Autodesk Fusion 360 part; units mm, degrees
(part 5 of 5)
sketch "Sketch1 (28)" plane through (0, 0, 0) normal (0, 0, 1) x (1, 0, 0) in component "main-switchbody (9)"
  line L0 (0, 0) -> (0, 20) construction
  line L1 (0, 20) -> (20, 20) construction
  line L2 (20, 20) -> (20, 0) construction
  line L3 (20, 0) -> (0, 0) construction
  line L4 (0, 0) -> (20, 20) construction
  line L5 (20, 0) -> (0, 20) construction
  line L6 (10, 0) -> (18.9, 0) construction
  line L7 (10, 10) -> (18.9, 10) construction
  line L8 (18.9, 10) -> (18.9, 18.9) construction
  line L9 (18.9, 18.9) -> (1.1, 18.9) construction
  line L10 (1.1, 18.9) -> (1.1, 1.1) construction
  line L11 (1.1, 1.1) -> (18.9, 1.1) construction
  line L12 (18.9, 1.1) -> (18.9, 18.9) construction
  line L13 (10, 10) -> (3.05, 10) construction
  line L14 (3.05, 10) -> (3.05, 16.95) construction
  line L15 (3.05, 16.95) -> (16.95, 16.95) construction
  line L16 (16.95, 16.95) -> (16.95, 3.05) construction
  line L17 (16.95, 3.05) -> (3.05, 3.05) construction
  line L18 (3.05, 3.05) -> (3.05, 16.95) construction
  line L19 (3.05, 3.05) -> (0, 3.05) construction
  line L20 (3.05, 3.05) -> (3.05, 0) construction
  line L21 (16.95, 3.05) -> (20, 3.05) construction
  line L22 (16.95, 16.95) -> (20, 16.95) construction
  line L23 (16.95, 16.95) -> (16.95, 20) construction
  line L24 (3.05, 16.95) -> (3.05, 20) construction
  line L25 (3.05, 16.95) -> (0, 16.95) construction
  line L26 (3.05, 18.9) -> (6.05, 18.9) construction
  line L27 (6.05, 18.9) -> (6.05, 20) construction
  line L28 (16.95, 18.9) -> (13.95, 18.9) construction
  line L29 (13.95, 18.9) -> (13.95, 20) construction
  line L30 (16.95, 3.05) -> (16.95, 0) construction
  line L31 (16.95, 1.1) -> (13.95, 1.1) construction
  line L32 (13.95, 1.1) -> (13.95, 0) construction
  line L33 (3.05, 1.1) -> (6.05, 1.1) construction
  line L34 (6.05, 1.1) -> (6.05, 0) construction
  line L35 (0, 20) -> (20, 20) construction
  line L36 (20, 20) -> (20, 0) construction
  line L37 (20, 0) -> (0, 0) construction
  line L38 (0, 0) -> (0, 20) construction
  line L39 (0, 20) -> (20, 20)
  line L40 (20, 20) -> (20, 0)
  line L41 (20, 0) -> (0, 0)
  line L42 (0, 0) -> (0, 20)
  line L43 (16.95, 3.05) -> (3.05, 3.05)
  line L44 (3.05, 3.05) -> (3.05, 16.95)
  line L45 (3.05, 16.95) -> (16.95, 16.95)
  line L46 (16.95, 16.95) -> (16.95, 3.05)
  line L47 (3.05, 1.1) -> (6.05, 1.1)
  line L48 (6.05, 1.1) -> (6.05, 0)
  line L49 (6.05, 0) -> (3.05, 0)
  line L50 (3.05, 0) -> (3.05, 1.1)
  line L51 (13.95, 1.1) -> (16.95, 1.1)
  line L52 (16.95, 1.1) -> (16.95, 0)
  line L53 (16.95, 0) -> (13.95, 0)
  line L54 (13.95, 0) -> (13.95, 1.1)
  line L55 (13.95, 20) -> (16.95, 20)
  line L56 (16.95, 20) -> (16.95, 18.9)
  line L57 (16.95, 18.9) -> (13.95, 18.9)
  line L58 (13.95, 18.9) -> (13.95, 20)
  line L59 (3.05, 20) -> (6.05, 20)
  line L60 (6.05, 20) -> (6.05, 18.9)
  line L61 (6.05, 18.9) -> (3.05, 18.9)
  line L62 (3.05, 18.9) -> (3.05, 20)
  line L63 (1.1, 10) -> (1.1, 12)
  line L64 (1.1, 10) -> (1.1, 8)
  line L65 (1.1, 8) -> (-1.9, 8)
  line L66 (-1.9, 8) -> (1.1, 8)
  line L67 (1.1, 8) -> (1.1, 12)
  line L68 (1.1, 12) -> (-1.9, 12)
  line L69 (-1.9, 12) -> (-1.9, 8)
  line L70 (3.05, 10) -> (3.05, 7.5) construction
  line L71 (3.05, 7.5) -> (2.55, 7.5) construction
  line L72 (2.55, 7.5) -> (2.55, 12.5) construction
  line L73 (2.55, 12.5) -> (3.05, 12.5085) construction
  line L74 (3.05, 12.5085) -> (3.05, 7.5) construction
  line L75 (2.55, 12.5) -> (16.95, 12.5) construction
  line L76 (16.95, 12.5) -> (17.45, 12.5) construction
  line L77 (17.45, 12.5) -> (17.45, 7.5) construction
  line L78 (17.45, 7.5) -> (16.95, 7.5) construction
  line L79 (16.95, 7.5) -> (16.95, 12.5) construction
  line L80 (17.45, 7.5) -> (16.95, 7.5)
  line L81 (16.95, 7.5) -> (16.95, 12.5)
  line L82 (16.95, 12.5) -> (17.45, 12.5)
  line L83 (17.45, 12.5) -> (17.45, 7.5)
  line L84 (3.05, 7.5) -> (2.55, 7.5)
  line L85 (2.55, 7.5) -> (2.55, 12.5)
  line L86 (2.55, 12.5) -> (3.05, 12.5)
  line L87 (3.05, 12.5) -> (3.05, 7.5)
  dimension "d1_9" = 20
  dimension "d2_9" = 20
  dimension "d3_9" = 8.9
  dimension "d4_9" = 8.9
  dimension "d5_9" = 8.9
  dimension "d6_9" = 17.8
  dimension "d7_9" = 17.8
  dimension "d8_9" = 6.95
  dimension "d9_9" = 6.95
  dimension "d10_9" = 13.9
  dimension "d11_9" = 13.9
  dimension "d12_9" = 13.9
  dimension "d13_9" = 3
  dimension "d14_9" = 3
  dimension "d15_9" = 3
  dimension "d16_9" = 3
  dimension "d21_15" = 3
  dimension "d58_15" = 2.5
  dimension "d59_15" = 0.5
  dimension "d60_15" = 5
  dimension "d61_15" = 0.5
  dimension "d62_15" = 5
  constraint coincident L0.start L3.end
  constraint vertical L0
  constraint perpendicular L0 L1
  constraint perpendicular L1 L2
  constraint perpendicular L0 L3
  constraint midpoint L3 L6.start
  constraint parallel L3 L6
  constraint midpoint L4 L7.start
  constraint parallel L6 L7
  constraint perpendicular L7 L8
  constraint perpendicular L8 L9
  constraint perpendicular L9 L10
  constraint coincident L5 L11.end
  constraint perpendicular L10 L11
  constraint perpendicular L12 L13
  constraint perpendicular L13 L14
  constraint perpendicular L14 L15
  constraint perpendicular L7 L16
  constraint perpendicular L16 L17
  constraint coincident L0 L19.end
  constraint perpendicular L0 L19
  constraint coincident L3 L20.end
  constraint perpendicular L3 L20
  constraint coincident L2 L21.end
  constraint perpendicular L2 L21
  constraint coincident L2 L22.end
  constraint perpendicular L2 L22
  constraint coincident L1 L23.end
  constraint perpendicular L1 L23
  constraint coincident L1 L24.end
  constraint perpendicular L1 L24
  constraint coincident L0 L25.end
  constraint perpendicular L0 L25
  constraint coincident L24 L26.start
  constraint coincident L9 L26.start
  constraint coincident L9 L26.end
  constraint coincident L1 L27.end
  constraint perpendicular L1 L27
  constraint coincident L9 L28.start
  constraint coincident L23 L28.start
  constraint perpendicular L23 L28
  constraint coincident L1 L29.end
  constraint perpendicular L1 L29
  constraint coincident L6 L30.end
  constraint coincident L30 L31.start
  constraint coincident L11 L31.start
  constraint perpendicular L30 L31
  constraint coincident L6 L32.end
  constraint coincident L11 L33.start
  constraint coincident L20 L33.start
  constraint perpendicular L20 L33
  constraint coincident L3 L34.end
  constraint perpendicular L3 L34
  constraint horizontal L35
  constraint vertical L36
  constraint horizontal L37
  constraint vertical L38
  constraint horizontal L39
  constraint vertical L40
  constraint horizontal L41
  constraint vertical L42
  constraint horizontal L43
  constraint vertical L44
  constraint horizontal L45
  constraint vertical L46
  constraint horizontal L47
  constraint vertical L48
  constraint horizontal L49
  constraint vertical L50
  constraint horizontal L51
  constraint vertical L52
  constraint horizontal L53
  constraint vertical L54
  constraint horizontal L55
  constraint vertical L56
  constraint horizontal L57
  constraint vertical L58
  constraint horizontal L59
  constraint vertical L60
  constraint horizontal L61
  constraint vertical L62
  constraint midpoint L10 L63.start
  constraint coincident L10 L63.end
  constraint parallel L10 L63
  constraint coincident L10 L64.end
  constraint perpendicular L0 L65
  constraint horizontal L66
  constraint vertical L67
  constraint horizontal L68
  constraint vertical L69
  constraint perpendicular L13 L70
  constraint perpendicular L70 L71
  constraint perpendicular L71 L72
  constraint coincident L14 L73.end
  constraint perpendicular L71 L74
  constraint coincident L16 L75.end
  constraint perpendicular L16 L75
  constraint perpendicular L16 L76
  constraint perpendicular L76 L77
  constraint coincident L16 L78.end
  constraint perpendicular L16 L78
  constraint horizontal L80
  constraint vertical L81
  constraint horizontal L82
  constraint vertical L83
  constraint horizontal L84
  constraint vertical L85
  constraint horizontal L86
  constraint vertical L87
  measures "d1_9" distance of L0.start L0.end
  measures "d2_9" distance of L0.end L1.end
  measures "d3_9" distance of L6.start L6.end
  measures "d4_9" distance of L7.start L7.end
  measures "d5_9" distance of L7.end L8.end
  measures "d6_9" distance of L8.end L9.end
  measures "d7_9" distance of L9.end L10.end
  measures "d8_9" distance of L7.start L13.end
  measures "d9_9" distance of L13.end L14.end
  measures "d10_9" distance of L14.end L15.end
  measures "d11_9" distance of L15.end L16.end
  measures "d12_9" distance of L16.end L17.end
  measures "d13_9" distance of L26.start L26.end
  measures "d14_9" distance of L28.start L28.end
  measures "d15_9" distance of L31.start L31.end
  measures "d16_9" distance of L33.start L33.end
  measures "d21_15" distance of L64.end L65.end
  measures "d58_15" distance of L13.end L70.end
  measures "d59_15" distance of L70.end L71.end
  measures "d60_15" distance of L71.end L72.end
  measures "d61_15" distance of L75.end L76.end
  measures "d62_15" distance of L76.end L77.end
extrude "Extrude3'''''''''''" add sketch "Sketch1 (28)" along normal blind 7.5 separate body contours L42 L63 L64 L65 L66 L67 L68 | L42 L65 L66 L68 L69 makes body 43 in component "main-switchbody (9)"
extrude "Extrude2'''''''''''" add sketch "Sketch1 (28)" along normal blind 4 separate body contours L39 L40 L41 L42 L47 L48 L50 L51 L52 L54 L56 L57 L58 L60 L61 L62 L63 L64 L65 L66 L67 L68 | L42 L63 L64 L65 L66 L67 L68 | L46 L80 L81 L82 L83 | L44 L84 L85 L86 L87 makes body 44 in component "main-switchbody (9)"
extrude "Extrude1'''''''''''''''''" add sketch "Sketch1 (28)" along normal blind 6 separate body contours L39 L59 L60 L61 L62 | L39 L55 L56 L57 L58 | L41 L47 L48 L49 L50 | L41 L51 L52 L53 L54 makes body 45 at (4.05, 1.1, 2) makes body 46 at (5.05, 20, 4) makes body 47 at (14.95, 1.1, 2) makes body 48 at (14.95, 20, 2) in component "main-switchbody (9)"
extrude "Extrude4'''''" cut sketch "Sketch1 (28)" along normal blind 2 contours L42 L65 L66 L68 L69 bodies 43 in component "main-switchbody (9)"
sketch "Sketch2 (22)" plane through (1.1, 0, 0) normal (1, 0, 0) x (0, 1, 0) in component "main-switchbody (9)"
  line L0 (8, 0) -> (12, 0)
  line L1 (12, 0) -> (12, 7.5)
  line L2 (12, 7.5) -> (8, 7.5)
  line L3 (8, 7.5) -> (8, 0)
  line L4 (8, 7.5) -> (8, 4) construction
  line L5 (8, 4) -> (12, 4) construction
  line L6 (12, 4) -> (12, 7.5) construction
  line L7 (12, 7.5) -> (8, 7.5) construction
  line L8 (8, 7.5) -> (8, 5.75) construction
  line L9 (8, 5.75) -> (12, 5.75) construction
  line L10 (8, 7.5) -> (12, 7.5)
  line L11 (12, 7.5) -> (12, 5.75)
  line L12 (12, 5.75) -> (8, 5.75)
  line L13 (8, 5.75) -> (8, 7.5)
  dimension "d26_15" = 1.75
  constraint coincident L2.end L3.start
  constraint coincident L3 L4.end
  constraint perpendicular L2 L4
  constraint coincident L1 L5.end
  constraint perpendicular L1 L5
  constraint coincident L1.end L2.start
  constraint perpendicular L2 L6
  constraint perpendicular L5 L8
  constraint midpoint L6 L9.end
  constraint horizontal L10
  constraint vertical L11
  constraint horizontal L12
  constraint vertical L13
  measures "d26_15" distance of L2.end L8.end
extrude "Extrude5'''''" add sketch "Sketch2 (22)" along normal blind 1 contours L1 L2 L3 L10 L11 L12 L13 bodies 43 in component "main-switchbody (9)"
extrude "Extrude6'''''" cut 1 faces at (-1.9, 10.6667, 3.8333) along direction (1, 0, 0) blind 1 on bodies 43 bodies 43 in component "main-switchbody (9)"
sketch "Sketch3 (6)" plane through (0, 18.9, 0) normal (0, -1, 0) x (1, 0, 0) in component "main-switchbody (9)"
  line L0 (3.05, 0) -> (6.05, 0)
  line L1 (6.05, 0) -> (6.05, 6)
  line L2 (6.05, 6) -> (3.05, 6)
  line L3 (3.05, 6) -> (3.05, 0)
  line L4 (3.05, 6) -> (3.05, 4) construction
  line L5 (6.05, 4) -> (6.05, 6) construction
  line L6 (3.05, 6) -> (3.05, 4.5) construction
  line L7 (6.05, 6) -> (6.05, 4.5) construction
  arc A0 (6.05, 4.5) -> (3.05, 4.5) centre (4.55, 4.5) ccw construction
  arc A1 (6.05, 4.5) -> (3.05, 4.5) centre (4.55, 4.5) ccw
  dimension "d31_15" = 1.5
  dimension "d32_15" = 1.5
  constraint coincident L2.end L3.start
  constraint coincident L3 L4.end
  constraint perpendicular L2 L4
  constraint coincident L1 L5.start
  constraint coincident L1.end L2.start
  constraint perpendicular L2 L5
  constraint perpendicular L2 L6
  constraint perpendicular L2 L7
  constraint tangent L2 A0
  constraint tangent L2 A1
  measures "d31_15" distance of L2.end L6.end
  measures "d32_15" distance of L1.end L7.end
extrude "Extrude7'''''" cut sketch "Sketch3 (6)" against normal blind 1.1 contours L2 L3 A1 | L1 L2 A1 bodies 46 in component "main-switchbody (9)"
sketch "Sketch4 (6)" plane through (0, 0, 0) normal (0, -1, 0) x (1, 0, 0) in component "main-switchbody (9)"
  line L0 (3.05, 0) -> (6.05, 0)
  line L1 (6.05, 0) -> (6.05, 6)
  line L2 (6.05, 6) -> (3.05, 6)
  line L3 (3.05, 6) -> (3.05, 0)
  line L4 (3.05, 6) -> (3.05, 4.5) construction
  line L5 (6.05, 6) -> (6.05, 4.5) construction
  arc A0 (6.05, 4.5) -> (3.05, 4.5) centre (4.55, 4.5) ccw
  constraint coincident L2.end L3.start
  constraint coincident L3 L4.end
  constraint perpendicular L2 L4
  constraint coincident L1.end L2.start
  constraint coincident L1 L5.end
  constraint perpendicular L2 L5
  constraint tangent L2 A0
extrude "Extrude8'''''" cut sketch "Sketch4 (6)" against normal blind 1.1 contours L2 L3 A0 | L1 L2 A0 bodies 45 in component "main-switchbody (9)"
sketch "Sketch5 (6)" plane through (0, 0, 0) normal (0, -1, 0) x (1, 0, 0) in component "main-switchbody (9)"
  line L0 (13.95, 0) -> (16.95, 0)
  line L1 (16.95, 0) -> (16.95, 6)
  line L2 (16.95, 6) -> (13.95, 6)
  line L3 (13.95, 6) -> (13.95, 0)
  line L4 (13.95, 6) -> (13.95, 4.5) construction
  line L5 (16.95, 6) -> (16.95, 4.5) construction
  arc A0 (16.95, 4.5) -> (13.95, 4.5) centre (15.45, 4.5) ccw
  constraint coincident L2.end L3.start
  constraint coincident L3 L4.end
  constraint perpendicular L2 L4
  constraint coincident L1.end L2.start
  constraint coincident L1 L5.end
  constraint perpendicular L2 L5
  constraint tangent L2 A0
extrude "Extrude9'''''" cut sketch "Sketch5 (6)" against normal blind 1.1 contours L2 L3 A0 | L1 L2 A0 bodies 47 in component "main-switchbody (9)"
sketch "Sketch6 (6)" plane through (0, 18.9, 0) normal (0, -1, 0) x (1, 0, 0) in component "main-switchbody (9)"
  line L0 (13.95, 0) -> (16.95, 0)
  line L1 (16.95, 0) -> (16.95, 6)
  line L2 (16.95, 6) -> (13.95, 6)
  line L3 (13.95, 6) -> (13.95, 0)
  line L4 (13.95, 6) -> (13.95, 4.5) construction
  line L5 (16.95, 6) -> (16.95, 4.5) construction
  arc A0 (16.95, 4.5) -> (13.95, 4.5) centre (15.45, 4.5) ccw
  constraint coincident L2.end L3.start
  constraint coincident L3 L4.end
  constraint perpendicular L2 L4
  constraint coincident L1.end L2.start
  constraint coincident L1 L5.end
  constraint perpendicular L2 L5
  constraint tangent L2 A0
extrude "Extrude10'''''" cut sketch "Sketch6 (6)" against normal blind 1.1 contours L2 L3 A0 | L1 L2 A0 bodies 48 in component "main-switchbody (9)"
sketch "Sketch7 (6)" plane through (0, 0, 4) normal (0, 0, 1) x (-1, 0, 0) in component "main-switchbody (9)"
  line L0 (-3.05, -16.95) -> (-16.95, -16.95)
  line L1 (-16.95, -16.95) -> (-16.95, -3.05)
  line L2 (-16.95, -3.05) -> (-3.05, -3.05)
  line L3 (-3.05, -3.05) -> (-3.05, -16.95)
  line L4 (-6.05, -20) -> (-6.05, -18.9)
  line L5 (-6.05, -18.9) -> (-3.05, -18.9)
  line L6 (-3.05, -18.9) -> (-3.05, -20)
  line L7 (-3.05, -20) -> (0, -20)
  line L8 (0, -20) -> (0, 0)
  line L9 (0, 0) -> (-3.05, 0)
  line L10 (-3.05, 0) -> (-3.05, -1.1)
  line L11 (-3.05, -1.1) -> (-6.05, -1.1)
  line L12 (-6.05, -1.1) -> (-6.05, 0)
  line L13 (-6.05, 0) -> (-13.95, 0)
  line L14 (-13.95, 0) -> (-13.95, -1.1)
  line L15 (-13.95, -1.1) -> (-16.95, -1.1)
  line L16 (-16.95, -1.1) -> (-16.95, 0)
  line L17 (-16.95, 0) -> (-20, 0)
  line L18 (-20, 0) -> (-20, -20)
  line L19 (-20, -20) -> (-16.95, -20)
  line L20 (-16.95, -20) -> (-16.95, -18.9)
  line L21 (-16.95, -18.9) -> (-13.95, -18.9)
  line L22 (-13.95, -18.9) -> (-13.95, -20)
  line L23 (-13.95, -20) -> (-6.05, -20)
  line L24 (-20, -10) -> (-20, -11.5) construction
  line L25 (-20, -10) -> (-20, -8.5) construction
  line L26 (-20, -8.5) -> (-19, -8.5) construction
  line L27 (-19, -8.5) -> (-19, -11.5) construction
  line L28 (-19, -11.5) -> (-20, -11.5) construction
  line L29 (-20, -11.5) -> (-21, -11.5) construction
  line L30 (-21, -11.5) -> (-21, -8.5) construction
  line L31 (-21, -8.5) -> (-20, -8.5) construction
  line L32 (-19, -11.5) -> (-21, -11.5)
  line L33 (-21, -11.5) -> (-21, -8.5)
  line L34 (-21, -8.5) -> (-19, -8.5)
  line L35 (-19, -8.5) -> (-19, -11.5)
  dimension "d41_15" = 1.5
  dimension "d42_15" = 1
  constraint midpoint L18 L24.start
  constraint parallel L18 L24
  constraint coincident L18 L25.end
  constraint parallel L18 L25
  constraint perpendicular L25 L26
  constraint perpendicular L26 L27
  constraint perpendicular L24 L29
  constraint perpendicular L29 L30
  constraint horizontal L32
  constraint vertical L33
  constraint horizontal L34
  constraint vertical L35
  measures "d41_15" distance of L24.start L24.end
  measures "d42_15" distance of L24.end L29.end
extrude "Extrude11'''''" add sketch "Sketch7 (6)" along normal blind 3 contours L18 L32 L33 L34 | L18 L32 L34 L35 bodies 44 in component "main-switchbody (9)"
extrude "Extrude12'''''" add 1 faces at (20, 8.5, 6) along direction (0, -1, 0) blind 0.5 on bodies 44 bodies 44 in component "main-switchbody (9)"
extrude "Extrude13'''''" add 1 faces at (20, 11.5, 6) along direction (0, 1, 0) blind 0.5 on bodies 44 bodies 44 in component "main-switchbody (9)"
extrude "Extrude14'''''" add 1 faces at (20.3333, 10.6667, 7) along direction (0, 0, 1) blind 0.75 on bodies 44 bodies 44 in component "main-switchbody (9)"
sketch "Sketch8 (6)" plane through (0, 0, 4) normal (0, 0, -1) x (1, 0, 0) in component "main-switchbody (9)"
  line L0 (20, -8) -> (20, -12)
  line L1 (20, -12) -> (21, -12)
  line L2 (21, -12) -> (21, -8)
  line L3 (21, -8) -> (20, -8)
  line L4 (20, -12) -> (20, -8)
  constraint coincident L0.end L1.start
  constraint coincident L0.start L3.end
extrude "Extrude15'''''" add sketch "Sketch8 (6)" along normal blind 2 bodies 44 in component "main-switchbody (9)"
sketch "Sketch9 (11)" plane through (19, 0, 0) normal (-1, 0, 0) x (0, -1, 0) in component "main-switchbody (9)"
  line L0 (-12, 4) -> (-8, 4)
  line L1 (-8, 4) -> (-8, 7.75)
  line L2 (-8, 7.75) -> (-12, 7.75)
  line L3 (-12, 7.75) -> (-12, 4)
  line L4 (-12, 7.75) -> (-12, 5.75) construction
  line L5 (-12, 5.75) -> (-8, 5.75) construction
  line L6 (-12, 7.75) -> (-8, 7.75)
  line L7 (-8, 7.75) -> (-8, 5.75)
  line L8 (-8, 5.75) -> (-12, 5.75)
  line L9 (-12, 5.75) -> (-12, 7.75)
  dimension "d53_15" = 2
  constraint coincident L2.end L3.start
  constraint perpendicular L2 L4
  constraint coincident L1 L5.end
  constraint perpendicular L1 L5
  constraint horizontal L6
  constraint vertical L7
  constraint horizontal L8
  constraint vertical L9
  measures "d53_15" distance of L2.end L4.end
extrude "Extrude16'''''" add sketch "Sketch9 (11)" along normal blind 0.5 contours L1 L2 L3 L6 L7 L8 L9 bodies 44 in component "main-switchbody (9)"
extrude "Extrude17'''''" cut 1 faces at (2.1, 9.3333, 6.9167) along direction (-1, 0, 0) blind 0.3 on bodies 43 bodies 43 in component "main-switchbody (9)"
extrude "Extrude18'''''" cut sketch "Sketch1 (28)" along normal blind 2.7 contours L44 L84 L85 L86 L87 bodies 44 in component "main-switchbody (9)"
extrude "Extrude19'''''" cut sketch "Sketch1 (28)" along normal blind 2.7 contours L46 L80 L81 L82 L83 bodies 44 in component "main-switchbody (9)"
extrude "Extrude20'''''" add sketch "Sketch1 (28)" against normal blind 0.2 contours L39 L40 L41 L42 L47 L48 L50 L51 L52 L54 L56 L57 L58 L60 L61 L62 L63 L64 L65 L66 L67 L68 | L39 L59 L60 L61 L62 | L42 L63 L64 L65 L66 L67 L68 | L39 L55 L56 L57 L58 | L41 L47 L48 L49 L50 | L41 L51 L52 L53 L54 bodies 43 44 45 46 47 48 in component "main-switchbody (9)"
fillet "Fillet1'''''" radius 1 2 edges at (21, 10, 7.75) (-0.9, 10, 7.5) on bodies 43 44 in component "main-switchbody (9)"
extrude "Extrude21'''''" add 1 faces at (2.8833, 9.1667, 2.7) along direction (0, 0, -1) blind 2.9 on bodies 43 bodies 43 in component "main-switchbody (9)"
extrude "Extrude22'''''" add 1 faces at (17.1167, 10.8333, 2.7) along direction (0, 0, -1) blind 2.9 on bodies 43 bodies 43 in component "main-switchbody (9)"
sketch "Sketch10 (6)" plane through (0, 0, 4) normal (0, 0, 1) x (-1, 0, 0) in component "main-switchbody (9)"
  line L0 (-3.05, -16.95) -> (-16.95, -16.95)
  line L1 (-16.95, -16.95) -> (-16.95, -3.05)
  line L2 (-16.95, -3.05) -> (-3.05, -3.05)
  line L3 (-3.05, -3.05) -> (-3.05, -16.95)
  line L4 (0, -12) -> (-1.1, -12)
  line L5 (-1.1, -12) -> (-1.1, -8)
  line L6 (-1.1, -8) -> (0, -8)
  line L7 (0, -8) -> (0, 0)
  line L8 (0, 0) -> (-3.05, 0)
  line L9 (-3.05, 0) -> (-3.05, -1.1)
  line L10 (-3.05, -1.1) -> (-6.05, -1.1)
  line L11 (-6.05, -1.1) -> (-6.05, 0)
  line L12 (-6.05, 0) -> (-13.95, 0)
  line L13 (-13.95, 0) -> (-13.95, -1.1)
  line L14 (-13.95, -1.1) -> (-16.95, -1.1)
  line L15 (-16.95, -1.1) -> (-16.95, 0)
  line L16 (-16.95, 0) -> (-20, 0)
  line L17 (-20, 0) -> (-20, -8)
  line L18 (-20, -8) -> (-19, -8)
  line L19 (-19, -8) -> (-19, -12)
  line L20 (-19, -12) -> (-20, -12)
  line L21 (-20, -12) -> (-20, -20)
  line L22 (-20, -20) -> (-16.95, -20)
  line L23 (-16.95, -20) -> (-16.95, -18.9)
  line L24 (-16.95, -18.9) -> (-13.95, -18.9)
  line L25 (-13.95, -18.9) -> (-13.95, -20)
  line L26 (-13.95, -20) -> (-6.05, -20)
  line L27 (-6.05, -20) -> (-6.05, -18.9)
  line L28 (-6.05, -18.9) -> (-3.05, -18.9)
  line L29 (-3.05, -18.9) -> (-3.05, -20)
  line L30 (-3.05, -20) -> (0, -20)
  line L31 (0, -20) -> (0, -12)
  line L32 (-3.05, -10) -> (-3.05, -12.5) construction
  line L33 (-3.05, -12.5) -> (-3.05, -7.5) construction
  line L34 (-3.05, -7.5) -> (-2.55, -7.5) construction
  line L35 (-2.55, -7.5) -> (-3.05, -7.5) construction
  line L36 (-3.05, -7.5) -> (-3.05, -12.5) construction
  line L37 (-3.05, -12.5) -> (-2.55, -12.5) construction
  line L38 (-2.55, -12.5) -> (-2.55, -7.5) construction
  line L39 (-3.05, -12.5) -> (-16.95, -12.5) construction
  line L40 (-16.95, -12.5) -> (-16.95, -7.5) construction
  line L41 (-16.95, -7.5) -> (-17.45, -7.5) construction
  line L42 (-17.45, -7.5) -> (-16.95, -7.5) construction
  line L43 (-16.95, -7.5) -> (-16.95, -12.5) construction
  line L44 (-16.95, -12.5) -> (-17.45, -12.5) construction
  line L45 (-17.45, -12.5) -> (-17.45, -7.5) construction
  line L46 (-16.95, -12.5) -> (-17.45, -12.5)
  line L47 (-17.45, -12.5) -> (-17.45, -7.5)
  line L48 (-17.45, -7.5) -> (-16.95, -7.5)
  line L49 (-16.95, -7.5) -> (-16.95, -12.5)
  line L50 (-2.55, -12.5) -> (-3.05, -12.5)
  line L51 (-3.05, -12.5) -> (-3.05, -7.5)
  line L52 (-3.05, -7.5) -> (-2.55, -7.5)
  line L53 (-2.55, -7.5) -> (-2.55, -12.5)
  dimension "d75_9" = 5
  dimension "d76_9" = 0.5
  dimension "d77_9" = 0.5
  constraint midpoint L3 L32.start
  constraint coincident L3 L32.end
  constraint perpendicular L0 L32
  constraint parallel L3 L33
  constraint perpendicular L33 L34
  constraint horizontal L35
  constraint vertical L36
  constraint horizontal L37
  constraint vertical L38
  constraint coincident L1 L39.end
  constraint perpendicular L1 L39
  constraint coincident L1 L40.end
  constraint perpendicular L39 L40
  constraint perpendicular L40 L41
  constraint horizontal L42
  constraint vertical L43
  constraint horizontal L44
  constraint vertical L45
  constraint horizontal L46
  constraint vertical L47
  constraint horizontal L48
  constraint vertical L49
  constraint horizontal L50
  constraint vertical L51
  constraint horizontal L52
  constraint vertical L53
  measures "d75_9" distance of L32.end L33.end
  measures "d76_9" distance of L33.end L34.end
  measures "d77_9" distance of L40.end L41.end
extrude "Extrude23'''''" cut sketch "Sketch10 (6)" against normal blind 2.9 contours L3 L50 L51 L52 L53 | L1 L46 L47 L48 L49 bodies 43 in component "main-switchbody (9)"
extrude "Extrude24'''''" cut 2 faces at (4.8122, 18.9, 5.1079) (15.1626, 18.9, 5.4316) along direction (0, 1, 0) blind 0.25 on bodies 43 bodies 43 in component "main-switchbody (9)"
extrude "Extrude25'''''" cut 2 faces at (4.2822, 1.1, 5.1824) (15.2673, 1.1, 4.9654) along direction (0, -1, 0) blind 0.25 on bodies 43 bodies 43 in component "main-switchbody (9)"
extrude "Extrude26'''''" add 1 faces at (1.0167, 12.3167, -0.2) along direction (0, 0, -1) blind 1 on bodies 43 bodies 43 in component "main-switchbody (9)"
extrude "Extrude27'''''" cut 1 faces at (1.0167, 12.3167, -1.2) along direction (0, 0, 1) blind 0.2 on bodies 43 bodies 43 in component "main-switchbody (9)"
extrude "Extrude28'''''" cut 2 faces at (17.1167, 10.8333, 1.1) (2.8833, 9.1667, 1.1) along direction (0, 0, -1) blind 0.8 on bodies 43 bodies 43 in component "main-switchbody (9)"
extrude "Extrude29'''''" cut 1 faces at (18.8333, 9.3333, 5.75) along direction (0, 0, 1) blind 0.2 on bodies 43 bodies 43 in component "main-switchbody (9)"
extrude "Extrude30'''''" cut 1 faces at (1.3333, 10.6667, 5.75) along direction (0, 0, 1) blind 0.2 on bodies 43 bodies 43 in component "main-switchbody (9)"
sketch "Sketch1 (29)" plane through (0, 0, 0.0152) normal (0, 0, -1) x (1, 0, 0) in component "mxledbit-switchbody v10 (9)"
  line L0 (4.5419, -16.2374) -> (4.5419, -2.3374)
  line L1 (4.5419, -2.3374) -> (18.4419, -2.3374)
  line L2 (18.4419, -2.3374) -> (18.4419, -16.2374)
  line L3 (18.4419, -16.2374) -> (4.5419, -16.2374)
  line L4 (1.4919, -19.2874) -> (21.4919, -19.2874)
  line L5 (21.4919, -19.2874) -> (21.4919, 0.7126)
  line L6 (21.4919, 0.7126) -> (1.4919, 0.7126)
  line L7 (1.4919, 0.7126) -> (1.4919, -19.2874)
ref_plane "WorkPlane1" through (5, 86.9951, 10.1395) normal (0, -0.997564, -0.069756) x (1, 0, 0) in component "wheel (5)"
sketch "Sketch2 (23)" plane through (5, 86.9951, 10.1395) normal (0, -0.997564, -0.069756) x (1, 0, 0) in component "wheel (5)"
  circle A0 centre (0, 0) radius 65
  dimension "d64_13" = 130
  constraint coincident A0.centre origin
  measures "d64_13" diameter of A0
component_pattern "component pattern'''''" in component "Pinky2"
sketch "Sketch2 (24)" plane through (0, 85.2823, 5.9635) normal (0, -0.997564, -0.069756) x (1, 0, 0) in component "IND-Sketch (5)"
  circle A0 centre (5, 4.0463) radius 65
  line L0 (5, 4.0463) -> (5, -60.9537) construction
  line L1 (5, -60.9537) -> (-38, -60.9537) construction
  line L2 (-38, -60.9537) -> (48, -60.9537)
  line L3 (48, -60.9537) -> (48, 4.0463)
  line L4 (48, 4.0463) -> (-38, 4.0463)
  line L5 (-38, 4.0463) -> (-38, -60.9537)
  dimension "d69_13" = 65
  dimension "d70_13" = 43
  dimension "d71_13" = 86
  dimension "d72_13" = 65
  constraint coincident A0.centre L0.start
  constraint vertical L0
  constraint perpendicular L0 L1
  constraint horizontal L2
  constraint vertical L3
  constraint horizontal L4
  constraint vertical L5
  measures "d69_13" distance of A0.centre L0.end
  measures "d70_13" distance of L0.end L1.end
  measures "d71_13" distance of L1.end L2.end
  measures "d72_13" distance of L1.end L4.end
sketch "Sketch9 (12)" plane through (5, 41.9534, 55.6343) normal (0, 0.573576, 0.819152) x (-1, 0, 0) in component "IND-Sketch (5)"
  line L0 (-45, -9.823) -> (5, -9.823) construction
  line L1 (-20, -9.823) -> (5, -9.823) construction
  line L2 (-20, -9.823) -> (-45, -9.823) construction
  circle A0 centre (-20, -9.823) radius 75 construction
  point P0 (-20, -9.823)
  point P1 (-45, -9.823)
  point P2 (5, -9.823)
  point P3 (5, -9.823)
  point P4 (-45, -9.823)
  dimension "d38_13" = 86
  dimension "d39_13" = 43
  dimension "d40_13" = 43
  dimension "d41_13" = 130
  constraint coincident P4 P1
  constraint horizontal L0
  constraint coincident P0 L1.start
  constraint parallel L0 L1
  constraint parallel L0 L2
sketch "Sketch1 (30)" plane through (0, 54.7581, -45.9475) normal (0, -0.766044, 0.642788) x (1, 0, 0) in component "IND-Sketch (5)"
  line L0 (-1.3269, 70.632) -> (-1.3269, 84.532)
  line L1 (-1.3269, 84.532) -> (12.5731, 84.532)
  line L2 (12.5731, 84.532) -> (12.5731, 70.632)
  line L3 (12.5731, 70.632) -> (-1.3269, 70.632)
  line L4 (-4.3769, 67.582) -> (15.6231, 67.582)
  line L5 (15.6231, 67.582) -> (15.6231, 87.582)
  line L6 (15.6231, 87.582) -> (-4.3769, 87.582)
  line L7 (-4.3769, 87.582) -> (-4.3769, 67.582)
  line L8 (-4.3769, 77.582) -> (15.6231, 77.582) construction
  line L9 (5.6231, 87.582) -> (5.6231, 67.582) construction
  point P0 (5.6231, 77.582)
  constraint midpoint L7 L8.start
  constraint midpoint L5 L8.end
  constraint midpoint L6 L9.start
  constraint midpoint L4 L9.end
  constraint midpoint L8 P0
component "Index1" placed x (0.983458, -0.041381, -0.176346) y (0.042188, 0.999109, 0.000831) z (0.176154, -0.008257, 0.984328) at (-2.2418, 1.6099, -4.6959)
component "Index2" placed x (0.984208, -0.02656, -0.175013) y (0.027095, 0.999633, 0.000664) z (0.174931, -0.005396, 0.984566) at (-2.4832, 0.1978, 1.0095)
component "Middle" placed x (0.984808, -0.015134, -0.172987) y (0.015134, 0.999885, -0.001319) z (0.172987, -0.001319, 0.984923) at (-10.562, 0.0958, 1.0948)
component "Ring" placed x (0.984808, 0, -0.173648) y (0, 1, 0) z (0.173648, 0, 0.984808) at (-3.6605, 0, -8.9798)
component "Pinky1" placed x (0.984658, -0.002254, -0.174482) y (0.001987, 0.999997, -0.001702) z (0.174485, 0.001329, 0.984659) at (10.2783, 2.1777, -23.775)
component "Pinky2" placed x (0.984658, -0.005299, -0.174416) y (0.005032, 0.999985, -0.001969) z (0.174424, 0.001061, 0.98467) at (9.9047, 3.203, -15.7658)
component "IND-Sketch" placed x (1, 0, 0) y (0, 1, 0) z (0, 0, 1) at (0, 0, 0) in component "Index1"
component "wheel" placed x (1, 0, 0) y (0, 1, 0) z (0, 0, 1) at (0, 0, 0) in component "Index1"
component "plug" placed x (1, 0, 0) y (0, 1, 0) z (0, 0, 1) at (0, 0, 0) in component "Index1"
component "plug" placed x (0.951017, -0.130647, -0.280173) y (0.130647, 0.991251, -0.018761) z (0.280173, -0.018761, 0.959766) at (-3.8633, 0.9283, 1.9908) in component "Index1"
component "plug" placed x (0.951017, 0.130647, 0.280173) y (-0.130647, 0.991251, -0.018761) z (-0.280173, -0.018761, 0.959766) at (4.3531, -0.3781, -0.8109) in component "Index1"
component "plug" placed x (0.808868, -0.248495, -0.5329) y (0.248495, 0.965863, -0.073208) z (0.5329, -0.073208, 0.843006) at (-6.8583, 2.3159, 4.9665) in component "Index1"
component "plug" placed x (0.808868, 0.248495, 0.5329) y (-0.248495, 0.965863, -0.073208) z (-0.5329, -0.073208, 0.843006) at (8.7696, -0.169, -0.3625) in component "Index1"
component "mxledbit-switchbody v10 (1)" placed x (1, 0, 0) y (0, -0.573576, -0.819152) z (0, 0.819152, -0.573576) at (-6, 30, 0) in component "plug"
component "main-switchbody (1)" placed x (1, 0, 0) y (0, 0.087156, -0.996195) z (0, 0.996195, 0.087156) at (1, 70.5187, 1.0257) in component "mxledbit-switchbody v10 (1)"
component "IND-Sketch (1)" placed x (1, 0, 0) y (0, 1, 0) z (0, 0, 1) at (0, 0, 0) in component "Index2"
component "wheel (1)" placed x (1, 0, 0) y (0, 1, 0) z (0, 0, 1) at (0, 0, 0) in component "Index2"
component "plug (1)" placed x (1, 0, 0) y (0, 1, 0) z (0, 0, 1) at (0, 0, 0) in component "Index2"
component "plug (1)" placed x (0.962425, -0.092875, -0.255171) y (0.092875, 0.995605, -0.012076) z (0.255171, -0.012076, 0.966821) at (-5.1501, 0.717, 1.9699) in component "Index2"
component "plug (1)" placed x (0.962425, 0.092875, 0.255171) y (-0.092875, 0.995605, -0.012076) z (-0.255171, -0.012076, 0.966821) at (5.5258, -0.2117, -0.5818) in component "Index2"
component "plug (1)" placed x (0.852525, -0.17877, -0.491165) y (0.17877, 0.982749, -0.047398) z (0.491165, -0.047398, 0.869776) at (-9.5374, 1.8854, 5.18) in component "Index2"
component "plug (1)" placed x (0.852525, 0.17877, 0.491165) y (-0.17877, 0.982749, -0.047398) z (-0.491165, -0.047398, 0.869776) at (11.0121, 0.0977, 0.2683) in component "Index2"
component "mxledbit-switchbody v10 (2)" placed x (1, 0, 0) y (0, -0.573576, -0.819152) z (0, 0.819152, -0.573576) at (-6, 30, 0) in component "plug (1)"
component "main-switchbody (2)" placed x (1, 0, 0) y (0, 0.258819, -0.965926) z (0, 0.965926, 0.258819) at (1, 66.4597, 26.6903) in component "mxledbit-switchbody v10 (2)"
component "IND-Sketch (2)" placed x (1, 0, 0) y (0, 1, 0) z (0, 0, 1) at (0, 0, 0) in component "Middle"
component "wheel (2)" placed x (1, 0, 0) y (0, 1, 0) z (0, 0, 1) at (0, 0, 0) in component "Middle"
component "plug (2)" placed x (1, 0, 0) y (0, 1, 0) z (0, 0, 1) at (0, 0, 0) in component "Middle"
component "plug (2)" placed x (0.966692, -0.022307, -0.25497) y (0.022307, 0.999747, -0.002892) z (0.25497, -0.002892, 0.966945) at (-3.7216, 0.1556, 1.7789) in component "Middle"
component "plug (2)" placed x (0.966692, 0.022307, 0.25497) y (-0.022307, 0.999747, -0.002892) z (-0.25497, -0.002892, 0.966945) at (4.0547, -0.0674, -0.7708) in component "Middle"
component "plug (2)" placed x (0.868986, -0.043128, -0.492954) y (0.043128, 0.999005, -0.011375) z (0.492954, -0.011375, 0.869981) at (-6.8621, 0.3891, 4.4475) in component "Middle"
component "plug (2)" placed x (0.868986, 0.043128, 0.492954) y (-0.043128, 0.999005, -0.011375) z (-0.492954, -0.011375, 0.869981) at (8.1723, -0.0422, -0.4821) in component "Middle"
component "mxledbit-switchbody v10 (3)" placed x (1, 0, 0) y (0, -0.573576, -0.819152) z (0, 0.819152, -0.573576) at (-6, 30, 0) in component "plug (2)"
component "main-switchbody (3)" placed x (1, 0, 0) y (0, 0.5, -0.866025) z (0, 0.866025, 0.5) at (1, 55.5969, 49.5501) in component "mxledbit-switchbody v10 (3)"
component "IND-Sketch (3)" placed x (1, 0, 0) y (0, 1, 0) z (0, 0, 1) at (0, 0, 0) in component "Ring"
component "wheel (3)" placed x (1, 0, 0) y (0, 1, 0) z (0, 0, 1) at (0, 0, 0) in component "Ring"
component "plug (3)" placed x (1, 0, 0) y (0, 1, 0) z (0, 0, 1) at (0, 0, 0) in component "Ring"
component "plug (3)" placed x (0.957285, 0, -0.289145) y (0, 1, 0) z (0.289145, 0, 0.957285) at (-2.6779, 0, 1.8729) in component "Ring"
component "plug (3)" placed x (0.957285, 0, 0.289145) y (0, 1, 0) z (-0.289145, 0, 0.957285) at (3.105, 0, -1.0186) in component "Ring"
component "plug (3)" placed x (0.832791, 0, -0.553588) y (0, 1, 0) z (0.553588, 0, 0.832791) at (-4.6998, 0, 4.44) in component "Ring"
component "plug (3)" placed x (0.832791, 0, 0.553588) y (0, 1, 0) z (-0.553588, 0, 0.832791) at (6.3719, 0, -1.0958) in component "Ring"
component "mxledbit-switchbody v10 (5)" placed x (1, 0, 0) y (0, -0.573576, -0.819152) z (0, 0.819152, -0.573576) at (-6, 30, 0) in component "plug (3)"
component "main-switchbody (5)" placed x (1, 0, 0) y (0, 0.573576, -0.819152) z (0, 0.819152, 0.573576) at (1, 35.8736, 62.963) in component "mxledbit-switchbody v10 (5)"
component "IND-Sketch (4)" placed x (1, 0, 0) y (0, 1, 0) z (0, 0, 1) at (0, 0, 0) in component "Pinky1"
component "wheel (4)" placed x (1, 0, 0) y (0, 1, 0) z (0, 0, 1) at (0, 0, 0) in component "Pinky1"
component "plug (4)" placed x (1, 0, 0) y (0, 1, 0) z (0, 0, 1) at (0, 0, 0) in component "Pinky1"
component "plug (4)" placed x (0.933528, 0.031246, -0.357141) y (-0.031246, 0.999495, 0.005771) z (0.357141, 0.005771, 0.934032) at (-1.0518, -0.1786, 2.0414) in component "Pinky1"
component "plug (4)" placed x (0.933528, -0.031246, 0.357141) y (0.031246, 0.999495, 0.005771) z (-0.357141, 0.005771, 0.934032) at (1.7166, 0.1339, -1.53) in component "Pinky1"
component "plug (4)" placed x (0.742947, 0.058338, -0.666803) y (-0.058338, 0.998047, 0.022318) z (0.666803, 0.022318, 0.7449) at (-1.2991, -0.3782, 4.3227) in component "Pinky1"
component "plug (4)" placed x (0.742947, -0.058338, 0.666803) y (0.058338, 0.998047, 0.022318) z (-0.666803, 0.022318, 0.7449) at (3.8697, 0.2052, -2.3453) in component "Pinky1"
component "mxledbit-switchbody v10 (7)" placed x (1, 0, 0) y (0, -0.573576, -0.819152) z (0, 0.819152, -0.573576) at (-6, 30, 0) in component "plug (4)"
component "main-switchbody (7)" placed x (1, 0, 0) y (0, 0.642788, -0.766044) z (0, 0.766044, 0.642788) at (1, 10.6994, 71.2959) in component "mxledbit-switchbody v10 (7)"
component "IND-Sketch (5)" placed x (1, 0, 0) y (0, 1, 0) z (0, 0, 1) at (0, 0, 0) in component "Pinky2"
component "wheel (5)" placed x (1, 0, 0) y (0, 1, 0) z (0, 0, 1) at (0, 0, 0) in component "Pinky2"
component "plug (5)" placed x (1, 0, 0) y (0, 1, 0) z (0, 0, 1) at (0, 0, 0) in component "Pinky2"
component "plug (5)" placed x (0.943267, 0.023162, -0.331227) y (-0.023162, 0.999724, 0.003948) z (0.331227, 0.003948, 0.943543) at (-1.0599, -0.1318, 1.8851) in component "Pinky2"
component "plug (5)" placed x (0.943267, -0.023162, 0.331227) y (0.023162, 0.999724, 0.003948) z (-0.331227, 0.003948, 0.943543) at (1.6272, 0.0998, -1.4271) in component "Pinky2"
component "plug (5)" placed x (0.779504, 0.043695, -0.624872) y (-0.043695, 0.998927, 0.015344) z (0.624872, 0.015344, 0.780577) at (-1.4321, -0.2807, 4.0144) in component "Pinky2"
component "plug (5)" placed x (0.779504, -0.043695, 0.624872) y (0.043695, 0.998927, 0.015344) z (-0.624872, 0.015344, 0.780577) at (3.6371, 0.1562, -2.2343) in component "Pinky2"
component "mxledbit-switchbody v10 (9)" placed x (1, 0, 0) y (0, -0.573576, -0.819152) z (0, 0.819152, -0.573576) at (-6, 30, 0) in component "plug (5)"
component "main-switchbody (9)" placed x (1, 0, 0) y (0, 0.62932, -0.777146) z (0, 0.777146, 0.62932) at (1, 3.613, 89.8638) in component "mxledbit-switchbody v10 (9)"
equation "IndexCircleDia = 140 mm" comment "Index1"
equation "IndexCircleLeanAngle = 120 deg" comment "Index1"
equation "d20 = IND_originX"
equation "d21 = IND_originY"
equation "IND_originX = 16 mm" comment "Index1"
equation "IND_originY = 16 mm" comment "Index1"
equation "IND_originZ = 10 mm" comment "Index1"
equation "d25 = IND_originY"
equation "d26 = IND_originZ"
equation "d27 = IND_originX"
equation "d28 = IND_originY"
equation "d29 = IND_originY"
equation "d30 = IND_originX"
equation "d31 = IndexCircleLeanAngle"
equation "d32 = IndexCircleDia"
equation "d33 = IND_originX / 2"
equation "d34 = IND_originX / 2"
equation "d35 = IND_originX / 2"
equation "d36 = IND_originX / 2"
equation "d37 = IND_originX / 2"
equation "d38 = IND_originX"
equation "d39 = IND_originX / 2"
equation "d40 = IND_originX / 2"
equation "d41 = IndexCircleDia"
equation "d42 = IndexCircleDia / 2"
equation "d43 = ( 13.9 / 2 ) * 1 mm"
equation "d44 = ( 13.9 / 2 ) * 1 mm"
equation "d45 = IndexCircleDia"
equation "d46 = IndexCircleDia / 2"
equation "d47 = IndexCircleDia"
equation "d51 = ( 13.9 / 2 ) * 1 mm"
equation "d52 = ( 13.9 / 2 ) * 1 mm"
equation "d55 = ( 13.9 / 2 ) * 1 mm - 2 mm"
equation "d57 = ( 13.9 / 2 ) * 1 mm - 2 mm"
equation "d64 = IndexCircleDia"
equation "d67 = IndexCircleOffsetDeg"
equation "IndexCircleOffsetDeg = 90 deg" comment "Index1"
equation "d69 = IndexCircleDia / 2"
equation "d70 = IND_originX / 2"
equation "d71 = IND_originX"
equation "d72 = IndexCircleDia / 2"
equation "IndexCircleDia_1 = 160 mm" comment "Index2"
equation "IndexCircleLeanAngle_1 = 110 deg" comment "Index2"
equation "d20_1 = IND_originX"
equation "d21_1 = IND_originY"
equation "IND_originX_1 = 30 mm" comment "Index2"
equation "IND_originY_1 = 30 mm" comment "Index2"
equation "IND_originZ_1 = 0 mm" comment "Index2"
equation "d25_1 = IND_originY_1"
equation "d26_1 = IND_originZ_1"
equation "d27_1 = IND_originX_1"
equation "d28_1 = IND_originY_1"
equation "d29_1 = IND_originY_1"
equation "d30_1 = IND_originX_1"
equation "d31_1 = IndexCircleLeanAngle_1"
equation "d32_1 = IndexCircleDia_1"
equation "d33_1 = IND_originX_1 / 2"
equation "d34_1 = IND_originX_1 / 2"
equation "d35_1 = IND_originX_1 / 2"
equation "d36_1 = IND_originX_1 / 2"
equation "d37_1 = IND_originX_1 / 2"
equation "d38_1 = IND_originX_1"
equation "d39_1 = IND_originX_1 / 2"
equation "d40_1 = IND_originX_1 / 2"
equation "d41_1 = IndexCircleDia_1"
equation "d42_1 = IndexCircleDia_1 / 2"
equation "d43_1 = ( 13.9 / 2 ) * 1 mm"
equation "d44_1 = ( 13.9 / 2 ) * 1 mm"
equation "d45_1 = IndexCircleDia_1"
equation "d46_1 = IndexCircleDia_1 / 2"
equation "d47_1 = IndexCircleDia_1"
equation "d51_1 = ( 13.9 / 2 ) * 1 mm"
equation "d52_1 = ( 13.9 / 2 ) * 1 mm"
equation "d55_1 = ( 13.9 / 2 ) * 1 mm - 2 mm"
equation "d57_1 = ( 13.9 / 2 ) * 1 mm - 2 mm"
equation "d64_1 = IndexCircleDia_1"
equation "d67_1 = IndexCircleOffsetDeg"
equation "IndexCircleOffsetDeg_1 = 90 deg" comment "Index2"
equation "d69_1 = IndexCircleDia_1 / 2"
equation "d70_1 = IND_originX_1 / 2"
equation "d71_1 = IND_originX_1"
equation "d72_1 = IndexCircleDia_1 / 2"
equation "IndexCircleDia_2 = 170 mm" comment "Middle"
equation "IndexCircleLeanAngle_2 = 95 deg" comment "Middle"
equation "d20_3 = IND_originX"
equation "d21_3 = IND_originY"
equation "IND_originX_2 = 34 mm" comment "Middle"
equation "IND_originY_2 = 34 mm" comment "Middle"
equation "IND_originZ_2 = 10 mm" comment "Middle"
equation "d25_3 = IND_originY_2"
equation "d26_3 = IND_originZ_2"
equation "d27_3 = IND_originX_2"
equation "d28_3 = IND_originY_2"
equation "d29_3 = IND_originY_2"
equation "d30_3 = IND_originX_2"
equation "d31_3 = IndexCircleLeanAngle_2"
equation "d32_3 = IndexCircleDia_2"
equation "d33_3 = IND_originX_2 / 2"
equation "d34_3 = IND_originX_2 / 2"
equation "d35_3 = IND_originX_2 / 2"
equation "d36_3 = IND_originX_2 / 2"
equation "d37_3 = IND_originX_2 / 2"
equation "d38_3 = IND_originX_2"
equation "d39_3 = IND_originX_2 / 2"
equation "d40_3 = IND_originX_2 / 2"
equation "d41_3 = IndexCircleDia_2"
equation "d42_3 = IndexCircleDia_2 / 2"
equation "d43_3 = ( 13.9 / 2 ) * 1 mm"
equation "d44_3 = ( 13.9 / 2 ) * 1 mm"
equation "d45_3 = IndexCircleDia_2"
equation "d46_3 = IndexCircleDia_2 / 2"
equation "d47_3 = IndexCircleDia_2"
equation "d51_3 = ( 13.9 / 2 ) * 1 mm"
equation "d52_3 = ( 13.9 / 2 ) * 1 mm"
equation "d55_3 = ( 13.9 / 2 ) * 1 mm - 2 mm"
equation "d57_3 = ( 13.9 / 2 ) * 1 mm - 2 mm"
equation "d64_3 = IndexCircleDia_2"
equation "d67_3 = IndexCircleOffsetDeg"
equation "IndexCircleOffsetDeg_2 = 90 deg" comment "Middle"
equation "d69_3 = IndexCircleDia_2 / 2"
equation "d70_3 = IND_originX_2 / 2"
equation "d71_3 = IND_originX_2"
equation "d72_3 = IndexCircleDia_2 / 2"
equation "IndexCircleDia_3 = 150 mm" comment "Ring"
equation "IndexCircleLeanAngle_3 = 90 deg" comment "Ring"
equation "d20_7 = IND_originX"
equation "d21_7 = IND_originY"
equation "IND_originX_3 = 49 mm" comment "Ring"
equation "IND_originY_3 = 49 mm" comment "Ring"
equation "IND_originZ_3 = 10 mm" comment "Ring"
equation "d25_7 = IND_originY_3"
equation "d26_7 = IND_originZ_3"
equation "d27_7 = IND_originX_3"
equation "d28_7 = IND_originY_3"
equation "d29_7 = IND_originY_3"
equation "d30_7 = IND_originX_3"
equation "d31_7 = IndexCircleLeanAngle_3"
equation "d32_7 = IndexCircleDia_3"
equation "d33_7 = IND_originX_3 / 2"
equation "d34_7 = IND_originX_3 / 2"
equation "d35_7 = IND_originX_3 / 2"
equation "d36_7 = IND_originX_3 / 2"
equation "d37_7 = IND_originX_3 / 2"
equation "d38_7 = IND_originX_3"
equation "d39_7 = IND_originX_3 / 2"
equation "d40_7 = IND_originX_3 / 2"
equation "d41_7 = IndexCircleDia_3"
equation "d42_7 = IndexCircleDia_3 / 2"
equation "d43_7 = ( 13.9 / 2 ) * 1 mm"
equation "d44_7 = ( 13.9 / 2 ) * 1 mm"
equation "d45_7 = IndexCircleDia_3"
equation "d46_7 = IndexCircleDia_3 / 2"
equation "d47_7 = IndexCircleDia_3"
equation "d51_7 = ( 13.9 / 2 ) * 1 mm"
equation "d52_7 = ( 13.9 / 2 ) * 1 mm"
equation "d55_7 = ( 13.9 / 2 ) * 1 mm - 2 mm"
equation "d57_7 = ( 13.9 / 2 ) * 1 mm - 2 mm"
equation "d64_7 = IndexCircleDia_3"
equation "d67_7 = IndexCircleOffsetDeg"
equation "IndexCircleOffsetDeg_3 = 90 deg" comment "Ring"
equation "d69_7 = IndexCircleDia_3 / 2"
equation "d70_7 = IND_originX_3 / 2"
equation "d71_7 = IND_originX_3"
equation "d72_7 = IndexCircleDia_3 / 2"
equation "IndexCircleDia_4 = 120 mm" comment "Pinky1"
equation "IndexCircleLeanAngle_4 = 85 deg" comment "Pinky1"
equation "d20_10 = IND_originX"
equation "d21_10 = IND_originY"
equation "IND_originX_4 = 65 mm" comment "Pinky1"
equation "IND_originY_4 = 65 mm" comment "Pinky1"
equation "IND_originZ_4 = 10 mm" comment "Pinky1"
equation "d25_10 = IND_originY_4"
equation "d26_10 = IND_originZ_4"
equation "d27_10 = IND_originX_4"
equation "d28_10 = IND_originY_4"
equation "d29_10 = IND_originY_4"
equation "d30_10 = IND_originX_4"
equation "d31_10 = IndexCircleLeanAngle_4"
equation "d32_10 = IndexCircleDia_4"
equation "d33_10 = IND_originX_4 / 2"
equation "d34_10 = IND_originX_4 / 2"
equation "d35_10 = IND_originX_4 / 2"
equation "d36_10 = IND_originX_4 / 2"
equation "d37_10 = IND_originX_4 / 2"
equation "d38_10 = IND_originX_4"
equation "d39_10 = IND_originX_4 / 2"
equation "d40_10 = IND_originX_4 / 2"
equation "d41_10 = IndexCircleDia_4"
equation "d42_10 = IndexCircleDia_4 / 2"
equation "d43_10 = ( 13.9 / 2 ) * 1 mm"
equation "d44_10 = ( 13.9 / 2 ) * 1 mm"
equation "d45_10 = IndexCircleDia_4"
equation "d46_10 = IndexCircleDia_4 / 2"
equation "d47_10 = IndexCircleDia_4"
equation "d51_10 = ( 13.9 / 2 ) * 1 mm"
equation "d52_10 = ( 13.9 / 2 ) * 1 mm"
equation "d55_10 = ( 13.9 / 2 ) * 1 mm - 2 mm"
equation "d57_10 = ( 13.9 / 2 ) * 1 mm - 2 mm"
equation "d64_10 = IndexCircleDia_4"
equation "d67_10 = IndexCircleOffsetDeg"
equation "IndexCircleOffsetDeg_4 = 90 deg" comment "Pinky1"
equation "d69_10 = IndexCircleDia_4 / 2"
equation "d70_10 = IND_originX_4 / 2"
equation "d71_10 = IND_originX_4"
equation "d72_10 = IndexCircleDia_4 / 2"
equation "IndexCircleDia_5 = 130 mm" comment "Pinky2"
equation "IndexCircleLeanAngle_5 = 86 deg" comment "Pinky2"
equation "d20_13 = IND_originX"
equation "d21_13 = IND_originY"
equation "IND_originX_5 = 86 mm" comment "Pinky2"
equation "IND_originY_5 = 85 mm" comment "Pinky2"
equation "IND_originZ_5 = 10 mm" comment "Pinky2"
equation "d25_13 = IND_originY_5"
equation "d26_13 = IND_originZ_5"
equation "d27_13 = IND_originX_5"
equation "d28_13 = IND_originY_5"
equation "d29_13 = IND_originY_5"
equation "d30_13 = IND_originX_5"
equation "d31_13 = IndexCircleLeanAngle_5"
equation "d32_13 = IndexCircleDia_5"
equation "d33_13 = IND_originX_5 / 2"
equation "d34_13 = IND_originX_5 / 2"
equation "d35_13 = IND_originX_5 / 2"
equation "d36_13 = IND_originX_5 / 2"
equation "d37_13 = IND_originX_5 / 2"
equation "d38_13 = IND_originX_5"
equation "d39_13 = IND_originX_5 / 2"
equation "d40_13 = IND_originX_5 / 2"
equation "d41_13 = IndexCircleDia_5"
equation "d42_13 = IndexCircleDia_5 / 2"
equation "d43_13 = ( 13.9 / 2 ) * 1 mm"
equation "d44_13 = ( 13.9 / 2 ) * 1 mm"
equation "d45_13 = IndexCircleDia_5"
equation "d46_13 = IndexCircleDia_5 / 2"
equation "d47_13 = IndexCircleDia_5"
equation "d51_13 = ( 13.9 / 2 ) * 1 mm"
equation "d52_13 = ( 13.9 / 2 ) * 1 mm"
equation "d55_13 = ( 13.9 / 2 ) * 1 mm - 2 mm"
equation "d57_13 = ( 13.9 / 2 ) * 1 mm - 2 mm"
equation "d64_13 = IndexCircleDia_5"
equation "d67_13 = IndexCircleOffsetDeg"
equation "IndexCircleOffsetDeg_5 = 90 deg" comment "Pinky2"
equation "d69_13 = IndexCircleDia_5 / 2"
equation "d70_13 = IND_originX_5 / 2"
equation "d71_13 = IND_originX_5"
equation "d72_13 = IndexCircleDia_5 / 2"
